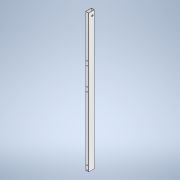
# Autodesk Inventor part: SP22V1 Tubo 40x80x1825mm
Saved by Autodesk Inventor 2021.2 (Build 252289000, 289)
## iProperties
Created: 2026-05-19
Part Number: SP22V1 Tubo 40x80x1825mm
Material: Acero, carbono
Document SubType Name: Modeling
Designer: nelso
Density: 7.85 g/cm^3
Appearance: Blanco
Author: nelso
Autodesk Inventor part; units mm, degrees
ref_plane "YZ Plane" through (0, 0, 0) normal (1, 0, 0) x (0, 1, 0)
ref_plane "XZ Plane" through (0, 0, 0) normal (0, 1, 0) x (-1, 0, 0)
ref_plane "XY Plane" through (0, 0, 0) normal (0, 0, 1) x (1, 0, 0)
sketch "Sketch1" plane through (0, 0, 0) normal (0, 1, 0) x (-1, 0, 0)
  line L0 (-20, 40) -> (20, 40)
  line L1 (20, 40) -> (20, -40)
  line L2 (20, -40) -> (-20, -40)
  line L3 (-20, -40) -> (-20, 40)
  line L4 (-20, 40) -> (20, -40) construction
  line L5 (20, 40) -> (-20, -40) construction
  line L6 (-17.76, 37.76) -> (17.76, 37.76)
  line L7 (17.76, 37.76) -> (17.76, -37.76)
  line L8 (17.76, -37.76) -> (-17.76, -37.76)
  line L9 (-17.76, -37.76) -> (-17.76, 37.76)
  line L10 (-17.76, 37.76) -> (17.76, -37.76) construction
  line L11 (17.76, 37.76) -> (-17.76, -37.76) construction
  point P0 (0, 0)
  dimension "d0" = 40
  dimension "d1" = 80
  dimension "d2" = 35.52
  dimension "d10" = 2.24
  constraints: 24 end point, 4 midpoint, 4 parallel, 2 horizontal, 2 perpendicular
  measures "d0" distance of L1.end L2.end
  measures "d1" distance of L0.end L1.end
  measures "d2" distance of L7.end L8.end
  measures "d10" distance between parallel lines of L2 L8
extrude "Extrusion1" add sketch "Sketch1" along normal blind 1824.7
fillet "Fillet1" radius 2 4 edges at (-17.76, 912.35, 37.76) (17.76, 912.35, -37.76) (17.76, 912.35, 37.76) (-17.76, 912.35, -37.76)
fillet "Fillet1" radius 4 4 edges at (20, 912.35, 40) (-20, 912.35, 40) (20, 912.35, -40) (-20, 912.35, -40)
sketch "Boceto3" plane through (-16, 0, 40) normal (0, 0, 1) x (1, 0, 0)
  circle A0 centre (16, 11.25) radius 4.5 projected
  circle A1 centre (16, 68.75) radius 4.5 projected
  circle A2 centre (16, 911.25) radius 4.5 projected
  circle A3 centre (16, 968.75) radius 4.5 projected
  circle A4 centre (16, 1268.75) radius 4.5 projected
  circle A5 centre (16, 1211.25) radius 4.5 projected
  circle A6 centre (16, 968.75) radius 5.5
  circle A7 centre (16, 911.25) radius 5.5
  circle A8 centre (16, 68.75) radius 5.5
  circle A9 centre (16, 11.25) radius 5.5
  circle A10 centre (16, 1268.75) radius 5.5
  circle A11 centre (16, 1211.25) radius 5.5
  point P0 (16, 0)
  dimension "d11" = 11
  dimension "d12" = 11
  dimension "d13" = 11
  dimension "d14" = 11
  dimension "d15" = 11
  dimension "d16" = 11
  constraints: 6 centre point, 6 coincident
  measures "d11" diameter of A6
  measures "d12" diameter of A7
  measures "d13" diameter of A8
  measures "d14" diameter of A9
  measures "d15" diameter of A10
  measures "d16" diameter of A11
extrude "Extrusión3" cut sketch "Boceto3" against normal blind 10 contours A0 | A1 | A2 | A3 | A4 | A5 | A6 | A7 | A8 | A9 | A10 | A11
sketch "Sketch8" plane through (20, 0, 36) normal (1, 0, 0) x (0, 0, -1)
  circle A0 centre (47.8654, 1771.4414) radius 11.11 projected
  point P0 (36, 0)
extrude "Extrusion7" cut sketch "Sketch8" against normal through all
body "Solid1"
